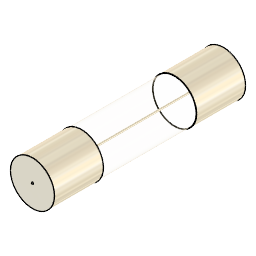
Fuse (Autodesk Fusion 360 design; units mm, degrees)
part number: 2025-09-30-14-32-08-949
part number: 2025-09-30-14-53-30-406
Autodesk Fusion 360 part; units mm, degrees
sketch "Sketch1" plane through (0, 0, 0) normal (0, 1, 0) x (1, 0, 0)
  circle A0 centre (0, 0) radius 2.25
  dimension "d1" = 4.5
  constraint coincident A0.centre origin
  measures "d1" diameter of A0
extrude "Extrude1" add sketch "Sketch1" along normal blind 5 makes body 1
sketch "Sketch2" plane through (0, 5, 0) normal (0, 1, 0) x (-1, 0, 0)
  circle A0 centre (0, 0) radius 2.25
  circle A1 centre (0, 0) radius 2.2
  dimension "d4" = 4.4
  constraint concentric A0 A1
  measures "d4" diameter of A1
extrude "Extrude2" add sketch "Sketch2" along normal blind 9.5 contours A1 bodies 1
sketch "Sketch3" plane through (0, 14.5, 0) normal (0, 1, 0) x (-1, 0, 0)
  circle A0 centre (0, 0) radius 2.2
  circle A1 centre (0, 0) radius 2.25
  dimension "d7" = 4.5
  constraint coincident A0.centre A1.centre
  measures "d7" diameter of A1
extrude "Extrude3" add sketch "Sketch3" along normal blind 5 separate body makes body 2
extrude "Extrude4" add 1 faces at (-0.5815, 14.5, -0.3062) along direction (0, 1, 0) blind 5 on bodies 1 bodies 1 2
sketch "Sketch4" plane through (0, 0, 0) normal (0, 1, 0) x (1, 0, 0)
  circle A0 centre (0, 0) radius 0.1
  dimension "d12" = 0.2
  constraint coincident A0.centre origin
  measures "d12" diameter of A0
extrude "Extrude5" add sketch "Sketch4" along normal blind 19.5 bodies 1
sketch "Sketch5" plane through (0, 0, 0) normal (0, 1, 0) x (1, 0, 0)
  circle A0 centre (0, 0) radius 0.1
  dimension "d15" = 0.2
  constraint coincident A0.centre origin
  measures "d15" diameter of A0
extrude "Extrude6" add sketch "Sketch5" along normal blind 19.5 bodies 1
sketch "Sketch6" plane through (0, 0, 0) normal (0, -1, 0) x (1, 0, 0)
  circle A0 centre (0, 0) radius 2.25
  circle A1 centre (0, 0) radius 0.25
  dimension "d18" = 0.5
  constraint coincident A0.centre A1.centre
  measures "d18" diameter of A1
extrude "Extrude7" add sketch "Sketch6" against normal blind 19.5 contours A1 bodies 1
sketch "Sketch7" plane through (0, 0, 0) normal (0, 1, 0) x (1, 0, 0)
  circle A0 centre (0, 0) radius 0.1
  dimension "d23" = 0.2
  constraint coincident A0.centre origin
  measures "d23" diameter of A0
extrude "Extrude1'" add sketch "Sketch7" along normal blind 19.5 separate body makes body 3 in component "Component"
component "Component" placed x (1, 0, 0) y (0, 1, 0) z (0, 0, 1) at (0, 0, 0)
